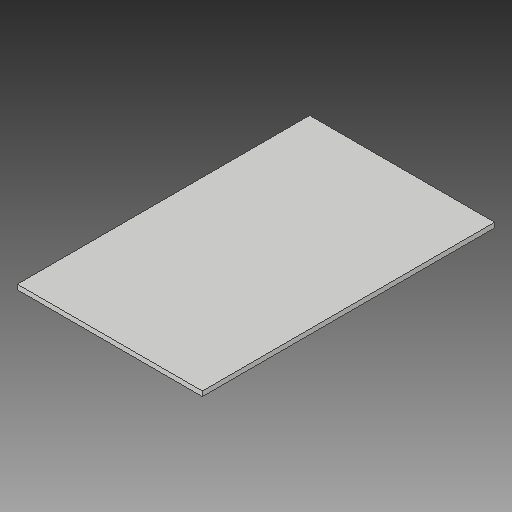
# Autodesk Inventor part: Cuerpo - Base
Saved by Autodesk Inventor 2019 (Build 230136000, 136)
## iProperties
Created: 2020-02-15
Part Number: Cuerpo - Base
Material: Genérico
Document SubType Name: Modeling
Designer: Mafer1
Density: 1 g/cm^3
Appearance: Valor por defecto
ancho_base: 120.000 mm
largo_base: 200.000 mm
Author: Mafer1
Autodesk Inventor part; units mm, degrees
ref_plane "YZ Plane" through (0, 0, 0) normal (1, 0, 0) x (0, 1, 0)
ref_plane "XZ Plane" through (0, 0, 0) normal (0, 1, 0) x (-1, 0, 0)
ref_plane "XY Plane" through (0, 0, 0) normal (0, 0, 1) x (1, 0, 0)
sketch "Boceto1" plane through (0, 0, 0) normal (0, 1, 0) x (-1, 0, 0)
  line L0 (0, 0) -> (126.6, 0)
  line L1 (126.6, 0) -> (126.6, -200)
  line L2 (126.6, -200) -> (0, -200)
  line L3 (0, -200) -> (0, 0)
  dimension "d0" = 200
  dimension "d1" = 126.6
  constraints: 8 end point, 2 parallel, 1 horizontal, 1 perpendicular
  measures "d0" distance of L0.end L1.end
  measures "d1" distance between parallel lines of L3 L1
extrude "Extrusión1" add sketch "Boceto1" along normal blind 3.3
equation "\"d0\" = largo_base"
equation "\"ancho_base\" = 120"
equation "\"largo_base\" = 200"
